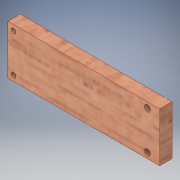
# Autodesk Inventor part: Sensor_Halterung_Teil2ipt
Saved by Autodesk Inventor 2018 (Build 220112000, 112)
## iProperties
Created: 2018-03-26
Part Number: Sensor_Halterung_Teil2ipt
Material: Holz (Eiche)
Document SubType Name: Modeling
Designer: Julian
Density: 0.76 g/cm^3
Appearance: Weißeiche - natur - mittlerer Glanz
Author: Julian
Autodesk Inventor part; units mm, degrees
ref_plane "YZ Plane" through (0, 0, 0) normal (1, 0, 0) x (0, 1, 0)
ref_plane "XZ Plane" through (0, 0, 0) normal (0, 1, 0) x (-1, 0, 0)
ref_plane "XY Plane" through (0, 0, 0) normal (0, 0, 1) x (1, 0, 0)
sketch "Skizze1" plane through (0, 0, 0) normal (0, 1, 0) x (-1, 0, 0)
  line L0 (0, 0) -> (59, 0)
  line L1 (59, 0) -> (59, -20)
  line L2 (59, -20) -> (0, -20)
  line L3 (0, -20) -> (0, 0)
  dimension "d0" = 59
  dimension "d1" = 20
  constraints: 8 end point, 2 parallel, 1 horizontal, 1 perpendicular
  measures "d0" distance of L1.end L2.end
  measures "d1" distance of L0.end L1.end
extrude "Extrusion1" add sketch "Skizze1" along normal blind 5
sketch "Skizze2" plane through (0, 5, 0) normal (0, 1, 0) x (1, 0, 0)
  point P0 (0, 0)
sketch "Skizze3" plane through (0, 5, 0) normal (0, 1, 0) x (1, 0, 0)
  line L0 (0, 0) -> (0, 20) projected
  line L1 (0, 0) -> (-2.5, 0)
  line L2 (-59, 0) -> (0, 0) projected
  line L3 (-2.5, 0) -> (-2.5, 2.25)
  line L4 (-2.5, 2.25) -> (-2.5, 17.75)
  dimension "d4" = 2.5
  dimension "d5" = 2.25
  dimension "d6" = 15.5
  constraints: 6 end point, 2 point on line, 1 perpendicular
  measures "d4" distance of L0.start L1.end
  measures "d5" distance of L1.end L3.end
  measures "d6" distance of L3.end L4.end
hole "Bohrung1" at (-2.5, 5, -2.25) at (-2.5, 5, -17.75) direction (0, -1, 0) diameter 2.5 end through all
sketch "Skizze4" plane through (0, 5, 0) normal (0, 1, 0) x (1, 0, 0)
  line L0 (-59, 0) -> (0, 0) projected
  line L1 (-58.751, 0) -> (-56.751, 0)
  line L2 (-56.751, 0) -> (-59.001, 0)
  line L3 (-56.751, 0) -> (-56.751, 2.25)
  line L4 (-56.751, 2.25) -> (-56.751, 17.75)
  dimension "d14" = 2
  dimension "d16" = 2.25
  dimension "d17" = 15.5
  constraints: 8 end point, 4 point on line, 1 vertical
  measures "d14" distance of L1.start L1.end
  measures "d16" distance of L1.end L3.end
  measures "d17" distance of L3.end L4.end
hole "Bohrung2" at (-56.751, 5, -2.25) at (-56.751, 5, -17.75) direction (0, -1, 0) diameter 2 end through all
sketch "Skizze5" plane through (0, 0, 0) normal (1, 0, 0) x (0, 0, -1)
  line L0 (20, 0) -> (0, 0) projected
  line L1 (0, 0) -> (20, 0)
  line L2 (20, 0) -> (20, 5)
  line L3 (20, 5) -> (0, 5)
  line L4 (0, 5) -> (0, 0)
  constraints: 8 end point, 2 parallel, 1 horizontal, 1 perpendicular
extrude "Extrusion2" add sketch "Skizze5" along normal blind 2.5
